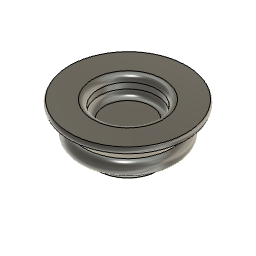
molde (Autodesk Fusion 360 design; units mm, degrees)
Autodesk Fusion 360 part; units mm, degrees
sketch "Boceto1" plane through (0, 0, 0) normal (0, 1, 0) x (1, 0, 0)
  arc A0 (75, -50) -> (75, -25) centre (70.8333, -37.5) ccw
  line L0 (75, -50) -> (100, -75)
  arc A1 (100, -85) -> (100, -75) centre (95, -80) ccw
  line L1 (100, -85) -> (50, -85)
  line L2 (50, -85) -> (50, -55)
  line L3 (50, -55) -> (0, -55)
  line L4 (0, -55) -> (0, 0)
  line L5 (-25, 0) -> (-25, -10)
  arc A2 (50, 0) -> (75, -25) centre (87.5, 12.5) ccw
  line L6 (50, 0) -> (0, 0)
  constraint coincident L4.end L6.end
  constraint tangent L0 A1
  constraint horizontal L1
  constraint perpendicular L1 L2
  constraint perpendicular L2 L3
  constraint perpendicular L3 L4
  constraint perpendicular L3 L5
  constraint tangent A0 A2
  constraint perpendicular L4 L6
revolve "Revolución1" add sketch "Boceto1" angle 360 about axis through (0, 0, 55) along (0, 0, -1) makes body 1
fillet "Empalme1" radius 10 1 edges at (-46.6164, -18.0808, 0) on bodies 1
fillet "Empalme2" radius 10 1 edges at (-46.6164, -18.0808, 85) on bodies 1
fillet "Empalme3" radius 10 1 edges at (-46.6164, -18.0808, 55) on bodies 1
sketch "Boceto7" plane through (0, 0, 0) normal (0, 0, 1) x (1, 0, 0)
  line L0 (150, -130) -> (-150, -130)
  line L1 (-150, -130) -> (-150, 130)
  line L2 (-150, 130) -> (150, 130)
  line L3 (150, 130) -> (150, -130)
  line L4 (150, -130) -> (-150, 130) construction
  line L5 (-150, -130) -> (150, 130) construction
  constraint horizontal L0
  constraint perpendicular L0 L1
  constraint parallel L0 L2
  constraint parallel L1 L3
  constraint coincident L4 origin
  constraint coincident L5 origin
extrude "Extruir1" add sketch "Boceto7" along normal blind 160 separate body makes body 2
combine "Combinar1" operation cut target body 2 tool bodies 1 keep tools
hidden bodies 2
